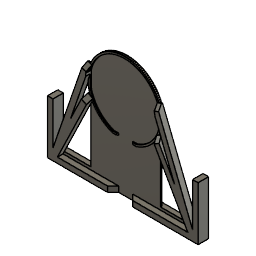
center_pass_wafer_jig (Autodesk Fusion 360 design; units mm, degrees)
part number: 2026-08-07-17-11-41-944
Autodesk Fusion 360 part; units mm, degrees
ref_plane "WorkPlane1" through (0, 0, 2) normal (0, 0, 1) x (1, 0, 0)
ref_plane "WorkPlane2" through (0, 0, 3.5) normal (0, 0, 1) x (1, 0, 0)
ref_plane "WorkPlane3" through (0, 0, 10) normal (0, 0, 1) x (1, 0, 0)
ref_plane "WorkPlane4" through (0, 0, 10.2) normal (0, 0, 1) x (1, 0, 0)
ref_plane "WorkPlane5" through (0, 0, 3.7) normal (0, 0, 1) x (1, 0, 0)
ref_plane "WorkPlane6" through (0, 0, -5) normal (0, 0, 1) x (1, 0, 0)
sketch "Center Nest Base Sketch" plane through (0, 0, 0) normal (0, 0, 1) x (1, 0, 0)
  line L0 (149.19, 109.35) -> (149.1396, 111.6618)
  line L1 (149.1396, 111.6618) -> (148.9883, 113.9693)
  line L2 (148.9883, 113.9693) -> (148.7366, 116.2679)
  line L3 (148.7366, 116.2679) -> (148.3848, 118.5534)
  line L4 (148.3848, 118.5534) -> (147.9337, 120.8213)
  line L5 (147.9337, 120.8213) -> (147.3841, 123.0674)
  line L6 (147.3841, 123.0674) -> (146.737, 125.2874)
  line L7 (146.737, 125.2874) -> (145.9937, 127.4771)
  line L8 (145.9937, 127.4771) -> (145.1556, 129.6322)
  line L9 (145.1556, 129.6322) -> (144.2243, 131.7488)
  line L10 (144.2243, 131.7488) -> (143.2016, 133.8227)
  line L11 (143.2016, 133.8227) -> (142.0893, 135.85)
  line L12 (142.0893, 135.85) -> (140.8897, 137.8269)
  line L13 (140.8897, 137.8269) -> (139.6051, 139.7496)
  line L14 (139.6051, 139.7496) -> (138.2377, 141.6144)
  line L15 (138.2377, 141.6144) -> (136.7904, 143.4177)
  line L16 (136.7904, 143.4177) -> (135.2657, 145.1563)
  line L17 (135.2657, 145.1563) -> (133.6667, 146.8267)
  line L18 (133.6667, 146.8267) -> (131.9963, 148.4257)
  line L19 (131.9963, 148.4257) -> (130.2577, 149.9504)
  line L20 (130.2577, 149.9504) -> (128.4544, 151.3977)
  line L21 (128.4544, 151.3977) -> (126.5896, 152.7651)
  line L22 (126.5896, 152.7651) -> (124.6669, 154.0497)
  line L23 (124.6669, 154.0497) -> (122.69, 155.2493)
  line L24 (122.69, 155.2493) -> (120.6627, 156.3616)
  line L25 (120.6627, 156.3616) -> (118.5888, 157.3843)
  line L26 (118.5888, 157.3843) -> (116.4722, 158.3156)
  line L27 (116.4722, 158.3156) -> (114.3171, 159.1537)
  line L28 (114.3171, 159.1537) -> (112.1274, 159.897)
  line L29 (112.1274, 159.897) -> (109.9074, 160.5441)
  line L30 (109.9074, 160.5441) -> (107.6613, 161.0937)
  line L31 (107.6613, 161.0937) -> (105.3934, 161.5448)
  line L32 (105.3934, 161.5448) -> (103.1079, 161.8966)
  line L33 (103.1079, 161.8966) -> (100.8093, 162.1483)
  line L34 (100.8093, 162.1483) -> (98.5018, 162.2996)
  line L35 (98.5018, 162.2996) -> (96.19, 162.35)
  line L36 (96.19, 162.35) -> (93.8782, 162.2996)
  line L37 (93.8782, 162.2996) -> (91.5707, 162.1483)
  line L38 (91.5707, 162.1483) -> (89.2721, 161.8966)
  line L39 (89.2721, 161.8966) -> (86.9866, 161.5448)
  line L40 (86.9866, 161.5448) -> (84.7187, 161.0937)
  line L41 (84.7187, 161.0937) -> (82.4726, 160.5441)
  line L42 (82.4726, 160.5441) -> (80.2526, 159.897)
  line L43 (80.2526, 159.897) -> (78.0629, 159.1537)
  line L44 (78.0629, 159.1537) -> (75.9078, 158.3156)
  line L45 (75.9078, 158.3156) -> (73.7912, 157.3843)
  line L46 (73.7912, 157.3843) -> (71.7173, 156.3616)
  line L47 (71.7173, 156.3616) -> (69.69, 155.2493)
  line L48 (69.69, 155.2493) -> (67.7131, 154.0497)
  line L49 (67.7131, 154.0497) -> (65.7904, 152.7651)
  line L50 (65.7904, 152.7651) -> (63.9256, 151.3977)
  line L51 (63.9256, 151.3977) -> (62.1223, 149.9504)
  line L52 (62.1223, 149.9504) -> (60.3837, 148.4257)
  line L53 (60.3837, 148.4257) -> (58.7133, 146.8267)
  line L54 (58.7133, 146.8267) -> (57.1143, 145.1563)
  line L55 (57.1143, 145.1563) -> (55.5896, 143.4177)
  line L56 (55.5896, 143.4177) -> (54.1423, 141.6144)
  line L57 (54.1423, 141.6144) -> (52.7749, 139.7496)
  line L58 (52.7749, 139.7496) -> (51.4903, 137.8269)
  line L59 (51.4903, 137.8269) -> (50.2907, 135.85)
  line L60 (50.2907, 135.85) -> (49.1784, 133.8227)
  line L61 (49.1784, 133.8227) -> (48.1557, 131.7488)
  line L62 (48.1557, 131.7488) -> (47.2244, 129.6322)
  line L63 (47.2244, 129.6322) -> (46.3863, 127.4771)
  line L64 (46.3863, 127.4771) -> (45.643, 125.2874)
  line L65 (45.643, 125.2874) -> (44.9959, 123.0674)
  line L66 (44.9959, 123.0674) -> (44.4463, 120.8213)
  line L67 (44.4463, 120.8213) -> (44.0067, 118.6111)
  line L68 (44.0067, 118.6111) -> (44.0067, 100.0889)
  line L69 (44.0067, 100.0889) -> (44.4463, 97.8787)
  line L70 (44.4463, 97.8787) -> (44.9959, 95.6326)
  line L71 (44.9959, 95.6326) -> (45.643, 93.4126)
  line L72 (45.643, 93.4126) -> (46.3863, 91.2229)
  line L73 (46.3863, 91.2229) -> (47.2244, 89.0678)
  line L74 (47.2244, 89.0678) -> (48.1557, 86.9512)
  line L75 (48.1557, 86.9512) -> (49.1784, 84.8773)
  line L76 (49.1784, 84.8773) -> (50.2907, 82.85)
  line L77 (50.2907, 82.85) -> (51.4903, 80.8731)
  line L78 (51.4903, 80.8731) -> (52.7749, 78.9504)
  line L79 (52.7749, 78.9504) -> (54.1423, 77.0856)
  line L80 (54.1423, 77.0856) -> (55.5896, 75.2823)
  line L81 (55.5896, 75.2823) -> (57.1143, 73.5437)
  line L82 (57.1143, 73.5437) -> (58.7133, 71.8733)
  line L83 (58.7133, 71.8733) -> (60.3837, 70.2743)
  line L84 (60.3837, 70.2743) -> (62.1223, 68.7496)
  line L85 (62.1223, 68.7496) -> (63.9256, 67.3023)
  line L86 (63.9256, 67.3023) -> (65.7904, 65.9349)
  line L87 (65.7904, 65.9349) -> (67.7131, 64.6503)
  line L88 (67.7131, 64.6503) -> (69.69, 63.4507)
  line L89 (69.69, 63.4507) -> (71.7173, 62.3384)
  line L90 (71.7173, 62.3384) -> (73.7912, 61.3157)
  line L91 (73.7912, 61.3157) -> (75.9078, 60.3844)
  line L92 (75.9078, 60.3844) -> (78.0629, 59.5463)
  line L93 (78.0629, 59.5463) -> (79.4828, 59.0643)
  line L94 (79.4828, 59.0643) -> (112.8972, 59.0643)
  line L95 (112.8972, 59.0643) -> (114.3171, 59.5463)
  line L96 (114.3171, 59.5463) -> (116.4722, 60.3844)
  line L97 (116.4722, 60.3844) -> (118.5888, 61.3157)
  line L98 (118.5888, 61.3157) -> (120.6627, 62.3384)
  line L99 (120.6627, 62.3384) -> (122.69, 63.4507)
  line L100 (122.69, 63.4507) -> (124.6669, 64.6503)
  line L101 (124.6669, 64.6503) -> (126.5896, 65.9349)
  line L102 (126.5896, 65.9349) -> (128.4544, 67.3023)
  line L103 (128.4544, 67.3023) -> (130.2577, 68.7496)
  line L104 (130.2577, 68.7496) -> (131.9963, 70.2743)
  line L105 (131.9963, 70.2743) -> (133.6667, 71.8733)
  line L106 (133.6667, 71.8733) -> (135.2657, 73.5437)
  line L107 (135.2657, 73.5437) -> (136.7904, 75.2823)
  line L108 (136.7904, 75.2823) -> (138.2377, 77.0856)
  line L109 (138.2377, 77.0856) -> (139.6051, 78.9504)
  line L110 (139.6051, 78.9504) -> (140.8897, 80.8731)
  line L111 (140.8897, 80.8731) -> (142.0893, 82.85)
  line L112 (142.0893, 82.85) -> (143.2016, 84.8773)
  line L113 (143.2016, 84.8773) -> (144.2243, 86.9512)
  line L114 (144.2243, 86.9512) -> (145.1556, 89.0678)
  line L115 (145.1556, 89.0678) -> (145.9937, 91.2229)
  line L116 (145.9937, 91.2229) -> (146.737, 93.4126)
  line L117 (146.737, 93.4126) -> (147.3841, 95.6326)
  line L118 (147.3841, 95.6326) -> (147.9337, 97.8787)
  line L119 (147.9337, 97.8787) -> (148.3848, 100.1466)
  line L120 (148.3848, 100.1466) -> (148.7366, 102.4321)
  line L121 (148.7366, 102.4321) -> (148.9883, 104.7307)
  line L122 (148.9883, 104.7307) -> (149.1396, 107.0382)
  line L123 (149.1396, 107.0382) -> (149.19, 109.35)
extrude "Center Nest Base" add sketch "Center Nest Base Sketch" along normal blind 2
sketch "100 mm Structural Sheet to Nest Centerline Sketch" plane through (0, 0, 0) normal (0, 0, 1) x (1, 0, 0)
  line L0 (46.19, -0.5) -> (146.19, -0.5)
  line L1 (146.19, -0.5) -> (146.19, 109.35)
  line L2 (146.19, 109.35) -> (46.19, 109.35)
  line L3 (46.19, 109.35) -> (46.19, -0.5)
extrude "100 mm Structural Sheet to Nest Centerline" add sketch "100 mm Structural Sheet to Nest Centerline Sketch" along normal blind 2
sketch "Center Nest Outer Wall Sketch" plane through (0, 0, 2) normal (0, 0, 1) x (1, 0, 0)
  line L0 (149.19, 109.35) -> (149.1396, 111.6618)
  line L1 (149.1396, 111.6618) -> (148.9883, 113.9693)
  line L2 (148.9883, 113.9693) -> (148.7366, 116.2679)
  line L3 (148.7366, 116.2679) -> (148.3848, 118.5534)
  line L4 (148.3848, 118.5534) -> (147.9337, 120.8213)
  line L5 (147.9337, 120.8213) -> (147.3841, 123.0674)
  line L6 (147.3841, 123.0674) -> (146.737, 125.2874)
  line L7 (146.737, 125.2874) -> (145.9937, 127.4771)
  line L8 (145.9937, 127.4771) -> (145.1556, 129.6322)
  line L9 (145.1556, 129.6322) -> (144.2243, 131.7488)
  line L10 (144.2243, 131.7488) -> (143.2016, 133.8227)
  line L11 (143.2016, 133.8227) -> (142.0893, 135.85)
  line L12 (142.0893, 135.85) -> (140.8897, 137.8269)
  line L13 (140.8897, 137.8269) -> (139.6051, 139.7496)
  line L14 (139.6051, 139.7496) -> (138.2377, 141.6144)
  line L15 (138.2377, 141.6144) -> (136.7904, 143.4177)
  line L16 (136.7904, 143.4177) -> (135.2657, 145.1563)
  line L17 (135.2657, 145.1563) -> (133.6667, 146.8267)
  line L18 (133.6667, 146.8267) -> (131.9963, 148.4257)
  line L19 (131.9963, 148.4257) -> (130.2577, 149.9504)
  line L20 (130.2577, 149.9504) -> (128.4544, 151.3977)
  line L21 (128.4544, 151.3977) -> (126.5896, 152.7651)
  line L22 (126.5896, 152.7651) -> (124.6669, 154.0497)
  line L23 (124.6669, 154.0497) -> (122.69, 155.2493)
  line L24 (122.69, 155.2493) -> (120.6627, 156.3616)
  line L25 (120.6627, 156.3616) -> (118.5888, 157.3843)
  line L26 (118.5888, 157.3843) -> (116.4722, 158.3156)
  line L27 (116.4722, 158.3156) -> (114.3171, 159.1537)
  line L28 (114.3171, 159.1537) -> (112.1274, 159.897)
  line L29 (112.1274, 159.897) -> (109.9074, 160.5441)
  line L30 (109.9074, 160.5441) -> (107.6613, 161.0937)
  line L31 (107.6613, 161.0937) -> (105.3934, 161.5448)
  line L32 (105.3934, 161.5448) -> (103.1079, 161.8966)
  line L33 (103.1079, 161.8966) -> (100.8093, 162.1483)
  line L34 (100.8093, 162.1483) -> (98.5018, 162.2996)
  line L35 (98.5018, 162.2996) -> (96.19, 162.35)
  line L36 (96.19, 162.35) -> (93.8782, 162.2996)
  line L37 (93.8782, 162.2996) -> (91.5707, 162.1483)
  line L38 (91.5707, 162.1483) -> (89.2721, 161.8966)
  line L39 (89.2721, 161.8966) -> (86.9866, 161.5448)
  line L40 (86.9866, 161.5448) -> (84.7187, 161.0937)
  line L41 (84.7187, 161.0937) -> (82.4726, 160.5441)
  line L42 (82.4726, 160.5441) -> (80.2526, 159.897)
  line L43 (80.2526, 159.897) -> (78.0629, 159.1537)
  line L44 (78.0629, 159.1537) -> (75.9078, 158.3156)
  line L45 (75.9078, 158.3156) -> (73.7912, 157.3843)
  line L46 (73.7912, 157.3843) -> (71.7173, 156.3616)
  line L47 (71.7173, 156.3616) -> (69.69, 155.2493)
  line L48 (69.69, 155.2493) -> (67.7131, 154.0497)
  line L49 (67.7131, 154.0497) -> (65.7904, 152.7651)
  line L50 (65.7904, 152.7651) -> (63.9256, 151.3977)
  line L51 (63.9256, 151.3977) -> (62.1223, 149.9504)
  line L52 (62.1223, 149.9504) -> (60.3837, 148.4257)
  line L53 (60.3837, 148.4257) -> (58.7133, 146.8267)
  line L54 (58.7133, 146.8267) -> (57.1143, 145.1563)
  line L55 (57.1143, 145.1563) -> (55.5896, 143.4177)
  line L56 (55.5896, 143.4177) -> (54.1423, 141.6144)
  line L57 (54.1423, 141.6144) -> (52.7749, 139.7496)
  line L58 (52.7749, 139.7496) -> (51.4903, 137.8269)
  line L59 (51.4903, 137.8269) -> (50.2907, 135.85)
  line L60 (50.2907, 135.85) -> (49.1784, 133.8227)
  line L61 (49.1784, 133.8227) -> (48.1557, 131.7488)
  line L62 (48.1557, 131.7488) -> (47.2244, 129.6322)
  line L63 (47.2244, 129.6322) -> (46.3863, 127.4771)
  line L64 (46.3863, 127.4771) -> (45.643, 125.2874)
  line L65 (45.643, 125.2874) -> (44.9959, 123.0674)
  line L66 (44.9959, 123.0674) -> (44.4463, 120.8213)
  line L67 (44.4463, 120.8213) -> (44.0067, 118.6111)
  line L68 (44.0067, 118.6111) -> (44.0067, 100.0889)
  line L69 (44.0067, 100.0889) -> (44.4463, 97.8787)
  line L70 (44.4463, 97.8787) -> (44.9959, 95.6326)
  line L71 (44.9959, 95.6326) -> (45.643, 93.4126)
  line L72 (45.643, 93.4126) -> (46.3863, 91.2229)
  line L73 (46.3863, 91.2229) -> (47.2244, 89.0678)
  line L74 (47.2244, 89.0678) -> (48.1557, 86.9512)
  line L75 (48.1557, 86.9512) -> (49.1784, 84.8773)
  line L76 (49.1784, 84.8773) -> (50.2907, 82.85)
  line L77 (50.2907, 82.85) -> (51.4903, 80.8731)
  line L78 (51.4903, 80.8731) -> (52.7749, 78.9504)
  line L79 (52.7749, 78.9504) -> (54.1423, 77.0856)
  line L80 (54.1423, 77.0856) -> (55.5896, 75.2823)
  line L81 (55.5896, 75.2823) -> (57.1143, 73.5437)
  line L82 (57.1143, 73.5437) -> (58.7133, 71.8733)
  line L83 (58.7133, 71.8733) -> (60.3837, 70.2743)
  line L84 (60.3837, 70.2743) -> (62.1223, 68.7496)
  line L85 (62.1223, 68.7496) -> (63.9256, 67.3023)
  line L86 (63.9256, 67.3023) -> (65.7904, 65.9349)
  line L87 (65.7904, 65.9349) -> (67.7131, 64.6503)
  line L88 (67.7131, 64.6503) -> (69.69, 63.4507)
  line L89 (69.69, 63.4507) -> (71.7173, 62.3384)
  line L90 (71.7173, 62.3384) -> (73.7912, 61.3157)
  line L91 (73.7912, 61.3157) -> (75.9078, 60.3844)
  line L92 (75.9078, 60.3844) -> (78.0629, 59.5463)
  line L93 (78.0629, 59.5463) -> (79.4828, 59.0643)
  line L94 (79.4828, 59.0643) -> (112.8972, 59.0643)
  line L95 (112.8972, 59.0643) -> (114.3171, 59.5463)
  line L96 (114.3171, 59.5463) -> (116.4722, 60.3844)
  line L97 (116.4722, 60.3844) -> (118.5888, 61.3157)
  line L98 (118.5888, 61.3157) -> (120.6627, 62.3384)
  line L99 (120.6627, 62.3384) -> (122.69, 63.4507)
  line L100 (122.69, 63.4507) -> (124.6669, 64.6503)
  line L101 (124.6669, 64.6503) -> (126.5896, 65.9349)
  line L102 (126.5896, 65.9349) -> (128.4544, 67.3023)
  line L103 (128.4544, 67.3023) -> (130.2577, 68.7496)
  line L104 (130.2577, 68.7496) -> (131.9963, 70.2743)
  line L105 (131.9963, 70.2743) -> (133.6667, 71.8733)
  line L106 (133.6667, 71.8733) -> (135.2657, 73.5437)
  line L107 (135.2657, 73.5437) -> (136.7904, 75.2823)
  line L108 (136.7904, 75.2823) -> (138.2377, 77.0856)
  line L109 (138.2377, 77.0856) -> (139.6051, 78.9504)
  line L110 (139.6051, 78.9504) -> (140.8897, 80.8731)
  line L111 (140.8897, 80.8731) -> (142.0893, 82.85)
  line L112 (142.0893, 82.85) -> (143.2016, 84.8773)
  line L113 (143.2016, 84.8773) -> (144.2243, 86.9512)
  line L114 (144.2243, 86.9512) -> (145.1556, 89.0678)
  line L115 (145.1556, 89.0678) -> (145.9937, 91.2229)
  line L116 (145.9937, 91.2229) -> (146.737, 93.4126)
  line L117 (146.737, 93.4126) -> (147.3841, 95.6326)
  line L118 (147.3841, 95.6326) -> (147.9337, 97.8787)
  line L119 (147.9337, 97.8787) -> (148.3848, 100.1466)
  line L120 (148.3848, 100.1466) -> (148.7366, 102.4321)
  line L121 (148.7366, 102.4321) -> (148.9883, 104.7307)
  line L122 (148.9883, 104.7307) -> (149.1396, 107.0382)
  line L123 (149.1396, 107.0382) -> (149.19, 109.35)
extrude "Center Nest Outer Wall" add sketch "Center Nest Outer Wall Sketch" along normal blind 1.5
sketch "Front Table Bar Sketch" plane through (0, 0, -5) normal (0, 0, 1) x (1, 0, 0)
  line L0 (-8, -12) -> (208, -12)
  line L1 (208, -12) -> (208, 0)
  line L2 (208, 0) -> (-8, 0)
  line L3 (-8, 0) -> (-8, -12)
extrude "Front Table Bar" add sketch "Front Table Bar Sketch" along normal blind 7
sketch "Left Full-Height Datum Bar Sketch" plane through (0, 0, -5) normal (0, 0, 1) x (1, 0, 0)
  line L0 (-8, -12) -> (0, -12)
  line L1 (0, -12) -> (0, 65)
  line L2 (0, 65) -> (-8, 65)
  line L3 (-8, 65) -> (-8, -12)
extrude "Left Full-Height Datum Bar" add sketch "Left Full-Height Datum Bar Sketch" along normal blind 15
sketch "Right Full-Height Datum Bar Sketch" plane through (0, 0, -5) normal (0, 0, 1) x (1, 0, 0)
  line L0 (200, -12) -> (208, -12)
  line L1 (208, -12) -> (208, 65)
  line L2 (208, 65) -> (200, 65)
  line L3 (200, 65) -> (200, -12)
extrude "Right Full-Height Datum Bar" add sketch "Right Full-Height Datum Bar Sketch" along normal blind 15
sketch "Continuous Front Top Rib Sketch" plane through (0, 0, 2) normal (0, 0, 1) x (1, 0, 0)
  line L0 (-8, -12) -> (208, -12)
  line L1 (208, -12) -> (208, -4)
  line L2 (208, -4) -> (-8, -4)
  line L3 (-8, -4) -> (-8, -12)
extrude "Continuous Front Top Rib" add sketch "Continuous Front Top Rib Sketch" along normal blind 8
sketch "Left Front Rib Lower Web Sketch" plane through (0, 0, 2) normal (0, 0, 1) x (1, 0, 0)
  line L0 (-3.6006, -6.2576) -> (43.5079, 91.0924)
  line L1 (43.5079, 91.0924) -> (50.709, 87.6076)
  line L2 (50.709, 87.6076) -> (3.6006, -9.7424)
  line L3 (3.6006, -9.7424) -> (-3.6006, -6.2576)
extrude "Left Front Rib Lower Web" add sketch "Left Front Rib Lower Web Sketch" along normal blind 1.5
sketch "Left Front Rib 45 Degree Thickness Taper Lower Sketch" plane through (0, 0, 3.5) normal (0, 0, 1) x (1, 0, 0)
  line L0 (-3.6006, -6.2576) -> (43.5079, 91.0924)
  line L1 (43.5079, 91.0924) -> (50.709, 87.6076)
  line L2 (50.709, 87.6076) -> (3.6006, -9.7424)
  line L3 (3.6006, -9.7424) -> (-3.6006, -6.2576)
sketch "Left Front Rib 45 Degree Thickness Taper Upper Sketch" plane through (0, 0, 10) normal (0, 0, 1) x (1, 0, 0)
  line L0 (-3.6006, -6.2576) -> (40.6765, 85.2414)
  line L1 (40.6765, 85.2414) -> (47.8777, 81.7567)
  line L2 (47.8777, 81.7567) -> (3.6006, -9.7424)
  line L3 (3.6006, -9.7424) -> (-3.6006, -6.2576)
loft "Left Front Rib 45 Degree Thickness Taper" add profiles "Left Front Rib 45 Degree Thickness Taper Lower Sketch", "Left Front Rib 45 Degree Thickness Taper Upper Sketch" section 1 section 2
sketch "Left Rear Rib Lower Web Sketch" plane through (0, 0, 2) normal (0, 0, 1) x (1, 0, 0)
  line L0 (-3.7836, -6.7023) -> (43.3248, 130.6477)
  line L1 (43.3248, 130.6477) -> (50.8921, 128.0523)
  line L2 (50.8921, 128.0523) -> (3.7836, -9.2977)
  line L3 (3.7836, -9.2977) -> (-3.7836, -6.7023)
extrude "Left Rear Rib Lower Web" add sketch "Left Rear Rib Lower Web Sketch" along normal blind 1.5
sketch "Left Rear Rib 45 Degree Thickness Taper Lower Sketch" plane through (0, 0, 3.5) normal (0, 0, 1) x (1, 0, 0)
  line L0 (-3.7836, -6.7023) -> (43.3248, 130.6477)
  line L1 (43.3248, 130.6477) -> (50.8921, 128.0523)
  line L2 (50.8921, 128.0523) -> (3.7836, -9.2977)
  line L3 (3.7836, -9.2977) -> (-3.7836, -6.7023)
sketch "Left Rear Rib 45 Degree Thickness Taper Upper Sketch" plane through (0, 0, 10) normal (0, 0, 1) x (1, 0, 0)
  line L0 (-3.7836, -6.7023) -> (41.216, 124.4993)
  line L1 (41.216, 124.4993) -> (48.7833, 121.9039)
  line L2 (48.7833, 121.9039) -> (3.7836, -9.2977)
  line L3 (3.7836, -9.2977) -> (-3.7836, -6.7023)
loft "Left Rear Rib 45 Degree Thickness Taper" add profiles "Left Rear Rib 45 Degree Thickness Taper Lower Sketch", "Left Rear Rib 45 Degree Thickness Taper Upper Sketch" section 1 section 2
sketch "Right Front Rib Lower Web Sketch" plane through (0, 0, 2) normal (0, 0, 1) x (1, 0, 0)
  line L0 (196.5132, -9.9602) -> (141.7848, 87.3898)
  line L1 (141.7848, 87.3898) -> (148.7583, 91.3102)
  line L2 (148.7583, 91.3102) -> (203.4868, -6.0398)
  line L3 (203.4868, -6.0398) -> (196.5132, -9.9602)
extrude "Right Front Rib Lower Web" add sketch "Right Front Rib Lower Web Sketch" along normal blind 1.5
sketch "Right Front Rib 45 Degree Thickness Taper Lower Sketch" plane through (0, 0, 3.5) normal (0, 0, 1) x (1, 0, 0)
  line L0 (196.5132, -9.9602) -> (141.7848, 87.3898)
  line L1 (141.7848, 87.3898) -> (148.7583, 91.3102)
  line L2 (148.7583, 91.3102) -> (203.4868, -6.0398)
  line L3 (203.4868, -6.0398) -> (196.5132, -9.9602)
sketch "Right Front Rib 45 Degree Thickness Taper Upper Sketch" plane through (0, 0, 10) normal (0, 0, 1) x (1, 0, 0)
  line L0 (196.5132, -9.9602) -> (144.9701, 81.7238)
  line L1 (144.9701, 81.7238) -> (151.9437, 85.6442)
  line L2 (151.9437, 85.6442) -> (203.4868, -6.0398)
  line L3 (203.4868, -6.0398) -> (196.5132, -9.9602)
loft "Right Front Rib 45 Degree Thickness Taper" add profiles "Right Front Rib 45 Degree Thickness Taper Lower Sketch", "Right Front Rib 45 Degree Thickness Taper Upper Sketch" section 1 section 2
sketch "Right Rear Rib Lower Web Sketch" plane through (0, 0, 2) normal (0, 0, 1) x (1, 0, 0)
  line L0 (196.2841, -9.4806) -> (141.5557, 127.8694)
  line L1 (141.5557, 127.8694) -> (148.9874, 130.8306)
  line L2 (148.9874, 130.8306) -> (203.7159, -6.5194)
  line L3 (203.7159, -6.5194) -> (196.2841, -9.4806)
extrude "Right Rear Rib Lower Web" add sketch "Right Rear Rib Lower Web Sketch" along normal blind 1.5
sketch "Right Rear Rib 45 Degree Thickness Taper Lower Sketch" plane through (0, 0, 3.5) normal (0, 0, 1) x (1, 0, 0)
  line L0 (196.2841, -9.4806) -> (141.5557, 127.8694)
  line L1 (141.5557, 127.8694) -> (148.9874, 130.8306)
  line L2 (148.9874, 130.8306) -> (203.7159, -6.5194)
  line L3 (203.7159, -6.5194) -> (196.2841, -9.4806)
sketch "Right Rear Rib 45 Degree Thickness Taper Upper Sketch" plane through (0, 0, 10) normal (0, 0, 1) x (1, 0, 0)
  line L0 (196.2841, -9.4806) -> (143.9617, 121.8311)
  line L1 (143.9617, 121.8311) -> (151.3935, 124.7923)
  line L2 (151.3935, 124.7923) -> (203.7159, -6.5194)
  line L3 (203.7159, -6.5194) -> (196.2841, -9.4806)
loft "Right Rear Rib 45 Degree Thickness Taper" add profiles "Right Rear Rib 45 Degree Thickness Taper Lower Sketch", "Right Rear Rib 45 Degree Thickness Taper Upper Sketch" section 1 section 2
sketch "Final Wafer Pocket Clearance Sketch" plane through (0, 0, 2) normal (0, 0, 1) x (1, 0, 0)
  line L0 (146.69, 109.35) -> (146.6419, 111.5528)
  line L1 (146.6419, 111.5528) -> (146.4978, 113.7514)
  line L2 (146.4978, 113.7514) -> (146.258, 115.9416)
  line L3 (146.258, 115.9416) -> (145.9228, 118.1192)
  line L4 (145.9228, 118.1192) -> (145.4929, 120.2802)
  line L5 (145.4929, 120.2802) -> (144.9693, 122.4204)
  line L6 (144.9693, 122.4204) -> (144.3527, 124.5356)
  line L7 (144.3527, 124.5356) -> (143.6445, 126.622)
  line L8 (143.6445, 126.622) -> (142.8459, 128.6755)
  line L9 (142.8459, 128.6755) -> (141.9585, 130.6922)
  line L10 (141.9585, 130.6922) -> (140.984, 132.6683)
  line L11 (140.984, 132.6683) -> (139.9243, 134.6)
  line L12 (139.9243, 134.6) -> (138.7813, 136.4836)
  line L13 (138.7813, 136.4836) -> (137.5572, 138.3156)
  line L14 (137.5572, 138.3156) -> (136.2543, 140.0925)
  line L15 (136.2543, 140.0925) -> (134.8752, 141.8108)
  line L16 (134.8752, 141.8108) -> (133.4225, 143.4673)
  line L17 (133.4225, 143.4673) -> (131.8989, 145.0589)
  line L18 (131.8989, 145.0589) -> (130.3073, 146.5825)
  line L19 (130.3073, 146.5825) -> (128.6508, 148.0352)
  line L20 (128.6508, 148.0352) -> (126.9325, 149.4143)
  line L21 (126.9325, 149.4143) -> (125.1556, 150.7172)
  line L22 (125.1556, 150.7172) -> (123.3236, 151.9413)
  line L23 (123.3236, 151.9413) -> (121.44, 153.0843)
  line L24 (121.44, 153.0843) -> (119.5083, 154.144)
  line L25 (119.5083, 154.144) -> (117.5322, 155.1185)
  line L26 (117.5322, 155.1185) -> (115.5155, 156.0059)
  line L27 (115.5155, 156.0059) -> (113.462, 156.8045)
  line L28 (113.462, 156.8045) -> (111.3756, 157.5127)
  line L29 (111.3756, 157.5127) -> (109.2604, 158.1293)
  line L30 (109.2604, 158.1293) -> (107.1202, 158.6529)
  line L31 (107.1202, 158.6529) -> (104.9592, 159.0828)
  line L32 (104.9592, 159.0828) -> (102.7816, 159.418)
  line L33 (102.7816, 159.418) -> (100.5914, 159.6578)
  line L34 (100.5914, 159.6578) -> (98.3928, 159.8019)
  line L35 (98.3928, 159.8019) -> (96.19, 159.85)
  line L36 (96.19, 159.85) -> (93.9872, 159.8019)
  line L37 (93.9872, 159.8019) -> (91.7886, 159.6578)
  line L38 (91.7886, 159.6578) -> (89.5984, 159.418)
  line L39 (89.5984, 159.418) -> (87.4208, 159.0828)
  line L40 (87.4208, 159.0828) -> (85.2598, 158.6529)
  line L41 (85.2598, 158.6529) -> (83.1196, 158.1293)
  line L42 (83.1196, 158.1293) -> (81.0044, 157.5127)
  line L43 (81.0044, 157.5127) -> (78.918, 156.8045)
  line L44 (78.918, 156.8045) -> (76.8645, 156.0059)
  line L45 (76.8645, 156.0059) -> (74.8478, 155.1185)
  line L46 (74.8478, 155.1185) -> (72.8717, 154.144)
  line L47 (72.8717, 154.144) -> (70.94, 153.0843)
  line L48 (70.94, 153.0843) -> (69.0564, 151.9413)
  line L49 (69.0564, 151.9413) -> (67.2244, 150.7172)
  line L50 (67.2244, 150.7172) -> (65.4475, 149.4143)
  line L51 (65.4475, 149.4143) -> (63.7292, 148.0352)
  line L52 (63.7292, 148.0352) -> (62.0727, 146.5825)
  line L53 (62.0727, 146.5825) -> (60.4811, 145.0589)
  line L54 (60.4811, 145.0589) -> (58.9575, 143.4673)
  line L55 (58.9575, 143.4673) -> (57.5048, 141.8108)
  line L56 (57.5048, 141.8108) -> (56.1257, 140.0925)
  line L57 (56.1257, 140.0925) -> (54.8228, 138.3156)
  line L58 (54.8228, 138.3156) -> (53.5987, 136.4836)
  line L59 (53.5987, 136.4836) -> (52.4557, 134.6)
  line L60 (52.4557, 134.6) -> (51.396, 132.6683)
  line L61 (51.396, 132.6683) -> (50.4215, 130.6922)
  line L62 (50.4215, 130.6922) -> (49.5341, 128.6755)
  line L63 (49.5341, 128.6755) -> (48.7355, 126.622)
  line L64 (48.7355, 126.622) -> (48.0273, 124.5356)
  line L65 (48.0273, 124.5356) -> (47.4107, 122.4204)
  line L66 (47.4107, 122.4204) -> (46.9067, 120.3604)
  line L67 (46.9067, 120.3604) -> (46.9067, 98.3396)
  line L68 (46.9067, 98.3396) -> (47.4107, 96.2796)
  line L69 (47.4107, 96.2796) -> (48.0273, 94.1644)
  line L70 (48.0273, 94.1644) -> (48.7355, 92.078)
  line L71 (48.7355, 92.078) -> (49.5341, 90.0245)
  line L72 (49.5341, 90.0245) -> (50.4215, 88.0078)
  line L73 (50.4215, 88.0078) -> (51.396, 86.0317)
  line L74 (51.396, 86.0317) -> (52.4557, 84.1)
  line L75 (52.4557, 84.1) -> (53.5987, 82.2164)
  line L76 (53.5987, 82.2164) -> (54.8228, 80.3844)
  line L77 (54.8228, 80.3844) -> (56.1257, 78.6075)
  line L78 (56.1257, 78.6075) -> (57.5048, 76.8892)
  line L79 (57.5048, 76.8892) -> (58.9575, 75.2327)
  line L80 (58.9575, 75.2327) -> (60.4811, 73.6411)
  line L81 (60.4811, 73.6411) -> (62.0727, 72.1175)
  line L82 (62.0727, 72.1175) -> (63.7292, 70.6648)
  line L83 (63.7292, 70.6648) -> (65.4475, 69.2857)
  line L84 (65.4475, 69.2857) -> (67.2244, 67.9828)
  line L85 (67.2244, 67.9828) -> (69.0564, 66.7587)
  line L86 (69.0564, 66.7587) -> (70.94, 65.6157)
  line L87 (70.94, 65.6157) -> (72.8717, 64.556)
  line L88 (72.8717, 64.556) -> (74.8478, 63.5815)
  line L89 (74.8478, 63.5815) -> (76.8645, 62.6941)
  line L90 (76.8645, 62.6941) -> (78.918, 61.8955)
  line L91 (78.918, 61.8955) -> (79.8937, 61.5643)
  line L92 (79.8937, 61.5643) -> (112.4863, 61.5643)
  line L93 (112.4863, 61.5643) -> (113.462, 61.8955)
  line L94 (113.462, 61.8955) -> (115.5155, 62.6941)
  line L95 (115.5155, 62.6941) -> (117.5322, 63.5815)
  line L96 (117.5322, 63.5815) -> (119.5083, 64.556)
  line L97 (119.5083, 64.556) -> (121.44, 65.6157)
  line L98 (121.44, 65.6157) -> (123.3236, 66.7587)
  line L99 (123.3236, 66.7587) -> (125.1556, 67.9828)
  line L100 (125.1556, 67.9828) -> (126.9325, 69.2857)
  line L101 (126.9325, 69.2857) -> (128.6508, 70.6648)
  line L102 (128.6508, 70.6648) -> (130.3073, 72.1175)
  line L103 (130.3073, 72.1175) -> (131.8989, 73.6411)
  line L104 (131.8989, 73.6411) -> (133.4225, 75.2327)
  line L105 (133.4225, 75.2327) -> (134.8752, 76.8892)
  line L106 (134.8752, 76.8892) -> (136.2543, 78.6075)
  line L107 (136.2543, 78.6075) -> (137.5572, 80.3844)
  line L108 (137.5572, 80.3844) -> (138.7813, 82.2164)
  line L109 (138.7813, 82.2164) -> (139.9243, 84.1)
  line L110 (139.9243, 84.1) -> (140.984, 86.0317)
  line L111 (140.984, 86.0317) -> (141.9585, 88.0078)
  line L112 (141.9585, 88.0078) -> (142.8459, 90.0245)
  line L113 (142.8459, 90.0245) -> (143.6445, 92.078)
  line L114 (143.6445, 92.078) -> (144.3527, 94.1644)
  line L115 (144.3527, 94.1644) -> (144.9693, 96.2796)
  line L116 (144.9693, 96.2796) -> (145.4929, 98.4198)
  line L117 (145.4929, 98.4198) -> (145.9228, 100.5808)
  line L118 (145.9228, 100.5808) -> (146.258, 102.7584)
  line L119 (146.258, 102.7584) -> (146.4978, 104.9486)
  line L120 (146.4978, 104.9486) -> (146.6419, 107.1472)
  line L121 (146.6419, 107.1472) -> (146.69, 109.35)
extrude "Final Wafer Pocket Clearance" cut sketch "Final Wafer Pocket Clearance Sketch" along normal blind 8.1
sketch "20 mm Front Bar Notch with 45 Degree Sides Lower Sketch" plane through (0, 0, 2) normal (0, 0, 1) x (1, 0, 0)
  line L0 (86.19, -12.1) -> (106.19, -12.1)
  line L1 (106.19, -12.1) -> (106.19, 0.1)
  line L2 (106.19, 0.1) -> (86.19, 0.1)
  line L3 (86.19, 0.1) -> (86.19, -12.1)
sketch "20 mm Front Bar Notch with 45 Degree Sides Upper Sketch" plane through (0, 0, 10.2) normal (0, 0, 1) x (1, 0, 0)
  line L0 (77.99, -20.3) -> (114.39, -20.3)
  line L1 (114.39, -20.3) -> (114.39, 8.3)
  line L2 (114.39, 8.3) -> (77.99, 8.3)
  line L3 (77.99, 8.3) -> (77.99, -20.3)
loft "20 mm Front Bar Notch with 45 Degree Sides" cut profiles "20 mm Front Bar Notch with 45 Degree Sides Lower Sketch", "20 mm Front Bar Notch with 45 Degree Sides Upper Sketch" section 1 section 2
sketch "20 mm Pickup Slot with 45 Degree Bevel Lower Sketch" plane through (0, 0, 2) normal (0, 0, 1) x (1, 0, 0)
  line L0 (86.19, 59.0643) -> (86.19, 62.0643)
  line L1 (86.19, 62.0643) -> (86.2756, 63.3696)
  line L2 (86.2756, 63.3696) -> (86.5307, 64.6525)
  line L3 (86.5307, 64.6525) -> (86.9512, 65.8911)
  line L4 (86.9512, 65.8911) -> (87.5297, 67.0643)
  line L5 (87.5297, 67.0643) -> (88.2565, 68.1519)
  line L6 (88.2565, 68.1519) -> (89.1189, 69.1354)
  line L7 (89.1189, 69.1354) -> (90.1024, 69.9978)
  line L8 (90.1024, 69.9978) -> (91.19, 70.7246)
  line L9 (91.19, 70.7246) -> (92.3632, 71.3031)
  line L10 (92.3632, 71.3031) -> (93.6018, 71.7236)
  line L11 (93.6018, 71.7236) -> (94.8847, 71.9787)
  line L12 (94.8847, 71.9787) -> (96.19, 72.0643)
  line L13 (96.19, 72.0643) -> (97.4953, 71.9787)
  line L14 (97.4953, 71.9787) -> (98.7782, 71.7236)
  line L15 (98.7782, 71.7236) -> (100.0168, 71.3031)
  line L16 (100.0168, 71.3031) -> (101.19, 70.7246)
  line L17 (101.19, 70.7246) -> (102.2776, 69.9978)
  line L18 (102.2776, 69.9978) -> (103.2611, 69.1354)
  line L19 (103.2611, 69.1354) -> (104.1235, 68.1519)
  line L20 (104.1235, 68.1519) -> (104.8503, 67.0643)
  line L21 (104.8503, 67.0643) -> (105.4288, 65.8911)
  line L22 (105.4288, 65.8911) -> (105.8493, 64.6525)
  line L23 (105.8493, 64.6525) -> (106.1044, 63.3696)
  line L24 (106.1044, 63.3696) -> (106.19, 62.0643)
  line L25 (106.19, 62.0643) -> (106.19, 59.0643)
  line L26 (106.19, 59.0643) -> (106.1044, 57.759)
  line L27 (106.1044, 57.759) -> (105.8493, 56.4761)
  line L28 (105.8493, 56.4761) -> (105.4288, 55.2375)
  line L29 (105.4288, 55.2375) -> (104.8503, 54.0643)
  line L30 (104.8503, 54.0643) -> (104.1235, 52.9767)
  line L31 (104.1235, 52.9767) -> (103.2611, 51.9932)
  line L32 (103.2611, 51.9932) -> (102.2776, 51.1308)
  line L33 (102.2776, 51.1308) -> (101.19, 50.404)
  line L34 (101.19, 50.404) -> (100.0168, 49.8255)
  line L35 (100.0168, 49.8255) -> (98.7782, 49.405)
  line L36 (98.7782, 49.405) -> (97.4953, 49.1499)
  line L37 (97.4953, 49.1499) -> (96.19, 49.0643)
  line L38 (96.19, 49.0643) -> (94.8847, 49.1499)
  line L39 (94.8847, 49.1499) -> (93.6018, 49.405)
  line L40 (93.6018, 49.405) -> (92.3632, 49.8255)
  line L41 (92.3632, 49.8255) -> (91.19, 50.404)
  line L42 (91.19, 50.404) -> (90.1024, 51.1308)
  line L43 (90.1024, 51.1308) -> (89.1189, 51.9932)
  line L44 (89.1189, 51.9932) -> (88.2565, 52.9767)
  line L45 (88.2565, 52.9767) -> (87.5297, 54.0643)
  line L46 (87.5297, 54.0643) -> (86.9512, 55.2375)
  line L47 (86.9512, 55.2375) -> (86.5307, 56.4761)
  line L48 (86.5307, 56.4761) -> (86.2756, 57.759)
  line L49 (86.2756, 57.759) -> (86.19, 59.0643)
sketch "20 mm Pickup Slot with 45 Degree Bevel Upper Sketch" plane through (0, 0, 3.7) normal (0, 0, 1) x (1, 0, 0)
  line L0 (84.49, 57.3643) -> (84.49, 63.7643)
  line L1 (84.49, 63.7643) -> (84.5901, 65.2915)
  line L2 (84.5901, 65.2915) -> (84.8887, 66.7925)
  line L3 (84.8887, 66.7925) -> (85.3806, 68.2417)
  line L4 (85.3806, 68.2417) -> (86.0575, 69.6143)
  line L5 (86.0575, 69.6143) -> (86.9078, 70.8868)
  line L6 (86.9078, 70.8868) -> (87.9169, 72.0374)
  line L7 (87.9169, 72.0374) -> (89.0675, 73.0465)
  line L8 (89.0675, 73.0465) -> (90.34, 73.8968)
  line L9 (90.34, 73.8968) -> (91.7126, 74.5737)
  line L10 (91.7126, 74.5737) -> (93.1618, 75.0656)
  line L11 (93.1618, 75.0656) -> (94.6628, 75.3642)
  line L12 (94.6628, 75.3642) -> (96.19, 75.4643)
  line L13 (96.19, 75.4643) -> (97.7172, 75.3642)
  line L14 (97.7172, 75.3642) -> (99.2182, 75.0656)
  line L15 (99.2182, 75.0656) -> (100.6674, 74.5737)
  line L16 (100.6674, 74.5737) -> (102.04, 73.8968)
  line L17 (102.04, 73.8968) -> (103.3125, 73.0465)
  line L18 (103.3125, 73.0465) -> (104.4631, 72.0374)
  line L19 (104.4631, 72.0374) -> (105.4722, 70.8868)
  line L20 (105.4722, 70.8868) -> (106.3225, 69.6143)
  line L21 (106.3225, 69.6143) -> (106.9994, 68.2417)
  line L22 (106.9994, 68.2417) -> (107.4913, 66.7925)
  line L23 (107.4913, 66.7925) -> (107.7899, 65.2915)
  line L24 (107.7899, 65.2915) -> (107.89, 63.7643)
  line L25 (107.89, 63.7643) -> (107.89, 57.3643)
  line L26 (107.89, 57.3643) -> (107.7899, 55.8371)
  line L27 (107.7899, 55.8371) -> (107.4913, 54.3361)
  line L28 (107.4913, 54.3361) -> (106.9994, 52.8869)
  line L29 (106.9994, 52.8869) -> (106.3225, 51.5143)
  line L30 (106.3225, 51.5143) -> (105.4722, 50.2418)
  line L31 (105.4722, 50.2418) -> (104.4631, 49.0911)
  line L32 (104.4631, 49.0911) -> (103.3125, 48.0821)
  line L33 (103.3125, 48.0821) -> (102.04, 47.2318)
  line L34 (102.04, 47.2318) -> (100.6674, 46.5549)
  line L35 (100.6674, 46.5549) -> (99.2182, 46.063)
  line L36 (99.2182, 46.063) -> (97.7172, 45.7644)
  line L37 (97.7172, 45.7644) -> (96.19, 45.6643)
  line L38 (96.19, 45.6643) -> (94.6628, 45.7644)
  line L39 (94.6628, 45.7644) -> (93.1618, 46.063)
  line L40 (93.1618, 46.063) -> (91.7126, 46.5549)
  line L41 (91.7126, 46.5549) -> (90.34, 47.2318)
  line L42 (90.34, 47.2318) -> (89.0675, 48.0821)
  line L43 (89.0675, 48.0821) -> (87.9169, 49.0911)
  line L44 (87.9169, 49.0911) -> (86.9078, 50.2418)
  line L45 (86.9078, 50.2418) -> (86.0575, 51.5143)
  line L46 (86.0575, 51.5143) -> (85.3806, 52.8869)
  line L47 (85.3806, 52.8869) -> (84.8887, 54.3361)
  line L48 (84.8887, 54.3361) -> (84.5901, 55.8371)
  line L49 (84.5901, 55.8371) -> (84.49, 57.3643)
loft "20 mm Pickup Slot with 45 Degree Bevel" cut profiles "20 mm Pickup Slot with 45 Degree Bevel Lower Sketch", "20 mm Pickup Slot with 45 Degree Bevel Upper Sketch" section 1 section 2
equation "tableWidth = 200.0 mm" comment "Nominal table width"
equation "insideStopSpan = 200.0 mm" comment "Exact inside span between table side datums"
equation "fieldCenterX = 96.19 mm" comment "Laser field center from table left"
equation "fieldCenterY = 109.35 mm" comment "Laser field center from table front"
equation "jigXCorrection = 0.0 mm" comment "Nest X calibration correction"
equation "jigYCorrection = 0.0 mm" comment "Nest Y calibration correction"
equation "baseThickness = 2.0 mm" comment "Wafer support base"
equation "sidewallHeight = 1.5 mm" comment "Wall above support base"
equation "strutWidth = 8.0 mm" comment "Constant rib width"
equation "strutHeight = 8.0 mm" comment "Rib height at frame"
equation "pickupGapWidth = 20.0 mm" comment "Primary-flat pickup opening"
